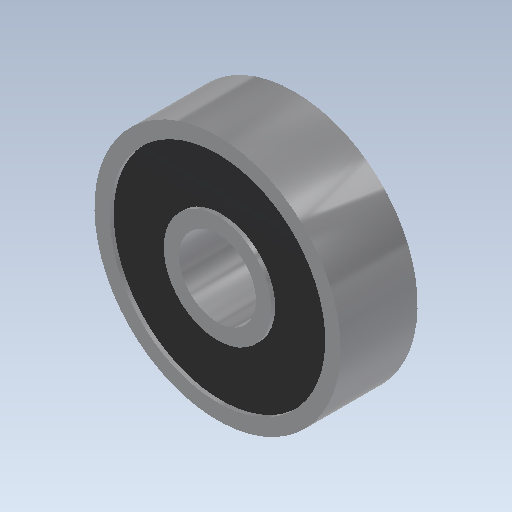
# Autodesk Inventor part: Ball Bearing 625 2RS 5x16x5
Saved by Autodesk Inventor 2022 (Build 260153000, 153)
## iProperties
Created: 2016-04-09
Part Number: Ball Bearing 625 2RS 5x16x5
Material: Generic
Document SubType Name: Modeling
Designer: Ben
Density: 1 g/cm^3
Appearance: Default
Author: Ben
Autodesk Inventor part; units mm, degrees
ref_plane "YZ Plane" through (0, 0, 0) normal (1, 0, 0) x (0, 1, 0)
ref_plane "XZ Plane" through (0, 0, 0) normal (0, 1, 0) x (-1, 0, 0)
ref_plane "XY Plane" through (0, 0, 0) normal (0, 0, 1) x (1, 0, 0)
sketch "Sketch1" plane through (0, 0, 0) normal (1, 0, 0) x (0, 1, 0)
  line L0 (0, 0) -> (0, 4.3483) construction
  line L1 (2.5, 0) -> (2.5, 5)
  line L2 (2.5, 5) -> (3.5, 5)
  line L3 (3.5, 5) -> (3.5, 4.75)
  line L4 (3.5, 4.75) -> (7, 4.75)
  line L5 (7, 4.75) -> (7, 5)
  line L6 (7, 5) -> (8, 5)
  line L7 (8, 5) -> (8, 0)
  line L8 (8, 0) -> (7, 0)
  line L9 (7, 0) -> (7, 0.25)
  line L10 (7, 0.25) -> (3.5, 0.25)
  line L11 (3.5, 0.25) -> (3.5, 0)
  line L12 (3.5, 0) -> (2.5, 0)
  line L13 (0, 0) -> (12.4665, 0) construction
  dimension "d0" = 5
  dimension "d1" = 16
  dimension "d2" = 1
  dimension "d3" = 1
  dimension "d4" = 0.25
  dimension "d5" = 0.25
  dimension "d6" = 5
  constraints: 28 end point, 7 collinear, 7 parallel, 4 perpendicular, 1 vertical
  measures "d0" diameter of L1 L0
  measures "d1" diameter of L7 L0
  measures "d2" distance between parallel lines of L1 L3
  measures "d3" distance between parallel lines of L7 L5
  measures "d4" distance between parallel lines of L2 L4
  measures "d5" distance between parallel lines of L12 L10
  measures "d6" distance between parallel lines of L8 L6
revolve "Revolution1" add sketch "Sketch1" angle 360 about axis through (0, 0, 0) along (0, 0, 1)
body "Solid1"
